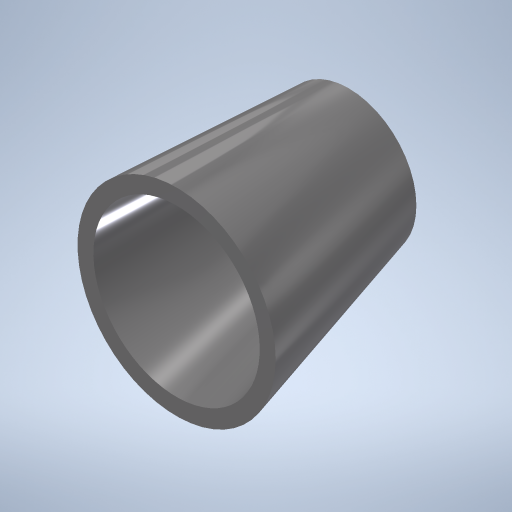
# Autodesk Inventor part: Redukcja asymetryczna Ø19x13x1,5 L=16,5
Saved by Autodesk Inventor 2023 (Build 270158000, 158)
## iProperties
RuleStatus: InUse
Created: 2022-03-21
Part Number: Redukcja asymetryczna Ø19x13x1,5 L=16,5
Material: 304
Description: Redukcja asymetryczna Ø19x13x1,5 L=16,5
Document SubType Name: Modelowanie
Designer: Radosław
Density: 8 g/cm^3
Sheet Metal Rule: 1,5
Sheet Metal Width: 0,000 mm
Sheet Metal Length: 0,000 mm
Sheet Metal Area: 0,000 mm^2
Appearance: Częściowo polerowany(1)
Author: Radosław
Autodesk Inventor part; units mm, degrees
ref_plane "YZ Plane" through (0, 0, 0) normal (1, 0, 0) x (0, 1, 0)
ref_plane "XY Plane" through (0, 0, 0) normal (0, 0, 1) x (1, 0, 0)
sketch "Szkic6" plane through (0, 0, 0) normal (0, 1, 0) x (-1, 0, 0)
  circle A0 centre (0, 0) radius 9.5
  dimension "d33" = 19
  constraints: 1 centre point, 1 coincident
  measures "d33" diameter of A0
ref_plane "Płaszczyzna konstrukcyjna1" through (0, 16.5, 0) normal (0, 1, 0) x (-1, 0, 0)
sketch "Szkic7" plane through (0, 16.5, 0) normal (0, 1, 0) x (-1, 0, 0)
  circle A0 centre (0, 3) radius 6.5
  line L0 (0, -20.3) -> (0, 20.3) construction
  circle A1 centre (0, 0) radius 9.5 construction
  dimension "d35" = 13
  constraints: 1 centre point, 1 coincident, 1 point on line, 1 tangent
  measures "d35" diameter of A0
loft "Wyciągnięcie złożone1" add profiles "Szkic6", "Szkic7"
shell "Skorupa1" thickness 1.5 removed faces 2 at (-3.8014, 16.5, 4.721) at (-2.3703, 0, -2.0999)
equation "\"d33\" = OD1"
equation "\"d35\" = OD2"
equation "\"d52\" = THK"
equation "\"SzerokośćGięciaPodcięcia\" = Grubość"
equation "\"RozmiarPodcięciaNarożnika\" = 4 * Grubość"
equation "\"PromieńPrzejścia\" = PromieńGięcia"
equation "\"Rozmiar_promienia_Jacobiego\" = PromieńGięcia"
equation "\"Wielk_odstępu\" = Grubość"
equation "\"d2\" = PromieńGięcia"
equation "\"d23\" = PromieńGięcia"
equation "\"OD1\" = 19"
equation "\"OD2\" = 13"
equation "\"L\" = 16.5"
equation "\"THK\" = 1.5"
equation "\"d34\" = L"
equation "\"Grubość\" = 1.5"
equation "\"PromieńGięcia\" = 3"
